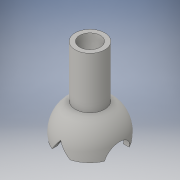
# Autodesk Inventor part: mcdave_caster
Saved by Autodesk Inventor 2016 (Build 200138000, 138)
## iProperties
Created: 2017-09-07
Part Number: mcdave_caster
Material: Generic
Document SubType Name: Modeling
Designer: student
Density: 1 g/cm^3
Appearance: Default
Author: student
Autodesk Inventor part; units mm, degrees
ref_plane "YZ Plane" through (0, 0, 0) normal (1, 0, 0) x (0, 1, 0)
ref_plane "XZ Plane" through (0, 0, 0) normal (0, 1, 0) x (-1, 0, 0)
ref_plane "XY Plane" through (0, 0, 0) normal (0, 0, 1) x (1, 0, 0)
sketch "Sketch1" plane through (0, 0, 0) normal (0, 0, 1) x (1, 0, 0)
  line L0 (0, 13.3294) -> (0, -14.3354)
  arc A0 (7.3657, -12.2179) -> (0, -2.6457) centre (0, -10.2657) ccw
  arc A1 (8.9332, -12.2179) -> (4.4666, -2.2868) centre (0, -10.2657) ccw
  line L1 (8.9332, -12.2179) -> (7.3657, -12.2179)
  line L2 (4.4666, -2.2868) -> (4.4666, 13.3294)
  line L3 (4.4666, 13.3294) -> (0, 13.3294)
  line L4 (0, 13.3294) -> (0, -2.6457)
  point P0 (0, 0)
  dimension "d0" = 15.24
  dimension "d1" = 1.524
  constraints: 10 end point, 4 point on circle, 2 centre point, 2 point on line, 2 vertical, 1 coincident, 1 collinear, 1 horizontal, 1 perpendicular
  measures "d0" diameter of A0
  measures "d1" radial gap between concentric circles of A1 A0
revolve "Revolution1" add sketch "Sketch1" angle 360 about axis through (0, 13.3294, 0) along (0, -1, 0)
sketch "Sketch2" plane through (0, 13.3294, 0) normal (0, 1, 0) x (1, 0, 0)
  circle A0 centre (0, 0) radius 3.1242
  dimension "d3" = 6.2484
  constraints: 1 centre point, 1 coincident
  measures "d3" diameter of A0
extrude "Extrusion1" cut sketch "Sketch2" against normal blind 7.62
sketch "Sketch3" plane through (0, 0, 0) normal (1, 0, 0) x (0, 1, 0)
  line L0 (-12.2179, 7.3657) -> (-12.2179, -7.3657) projected
  circle A0 centre (-12.2179, 0) radius 3.7062
  point P0 (0, 0)
  constraints: 1 centre point, 1 midpoint
extrude "Extrusion2" cut sketch "Sketch3" along normal mid plane 101.6
sketch "Sketch4" plane through (0, 0, 0) normal (0, 0, 1) x (1, 0, 0)
  line L0 (-8.1281, -12.2179) -> (8.1281, -12.2179) projected
  line L1 (0, -12.2179) -> (0, -8.1441)
  line L2 (0, -8.1441) -> (-3.0698, -12.2179)
  line L3 (0, -8.1441) -> (5.1009, -8.1441) construction
  line L4 (0, -8.1441) -> (2.5504, -12.2179)
  point P0 (0, 0)
  dimension "d8" = 127
  constraints: 8 end point, 2 point on line, 1 equal length, 1 horizontal, 1 midpoint, 1 vertical
  measures "d8" angle of L2 L3
extrude "Extrusion3" cut sketch "Sketch4" along normal mid plane 101.6
body "Solid1"
